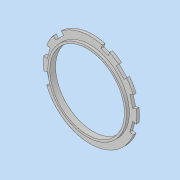
# Autodesk Inventor part: BallastTankMillOutline
Saved by Autodesk Inventor 2017.3 (Build 213256000, 256)
## iProperties
Created: 2018-07-14
Part Number: BallastTankMillOutline
Material: Generic
Document SubType Name: Modeling
Designer: Derek Wider
Density: 1 g/cm^3
Appearance: Default
Author: Derek Wider
Autodesk Inventor part; units mm, degrees
ref_plane "YZ Plane" through (0, 0, 0) normal (1, 0, 0) x (0, 1, 0)
ref_plane "XZ Plane" through (0, 0, 0) normal (0, 1, 0) x (-1, 0, 0)
ref_plane "XY Plane" through (0, 0, 0) normal (0, 0, 1) x (1, 0, 0)
sketch "Sketch1" plane through (0, 0, 0) normal (0, 0, 1) x (1, 0, 0)
  circle A0 centre (0, 0) radius 34.798
  circle A1 centre (0, 0) radius 41.275
  line L0 (38.2986, -15.3898) -> (35.2745, -14.5795)
  line L1 (35.2745, -14.5795) -> (37.8384, -5.011)
  line L2 (37.8384, -5.011) -> (40.8624, -5.8213)
  line L3 (0, 0) -> (36.5564, -9.7953) construction
  line L4 (0, 0) -> (34.798, 0) construction
  line L5 (36.5564, -9.7953) -> (39.8686, -10.6828) construction
  dimension "d0" = 69.596
  dimension "d1" = 82.55
  dimension "d2" = 15
  dimension "d3" = 9.906
  dimension "d4" = 3.429
  constraints: 12 end point, 3 point on circle, 2 coincident, 2 parallel, 1 centre point, 1 horizontal, 1 horizontal alignment, 1 midpoint, 1 perpendicular, 2 other
  measures "d1" diameter of A1
  measures "d2" angle of L3 L4
  measures "d3" distance between parallel lines of L0 L2
  measures "d4" distance of L3.end L5.end
extrude "Extrusion1" add sketch "Sketch1" along normal blind 2.54
extrude "Extrusion2" cut sketch "Sketch1" along normal blind 2.54 contours L0 L1 L2 A1 picked at (37.7926, -9.5555)
pattern_circular "Circular Pattern1" count 3 over 60 about axis through (0, 0, 0) along (0, 0, 1) of "Extrusion2"
mirror "Mirror1" about plane through (0, 0, 0) normal (1, 0, 0) of "Extrusion2", "Circular Pattern1"
sketch "Sketch2" plane through (0, 0, 0) normal (0, 0, -1) x (-1, 0, 0)
  circle A0 centre (0, 0) radius 34.798 projected
  circle A1 centre (0, 0) radius 33.02
  dimension "d12" = 66.04
  constraints: 1 centre point, 1 coincident
  measures "d12" diameter of A1
extrude "Extrusion3" add sketch "Sketch2" against normal blind 5.08
sketch "Sketch3" plane through (0, 0, 0) normal (0, 0, -1) x (-1, 0, 0)
  arc A0 (25.4726, 32.4772) -> (-25.4726, 32.4772) centre (0, 0) ccw projected
  line L0 (-17.2903, 37.4789) -> (-16.1691, 34.3986)
  line L1 (-16.1691, 34.3986) -> (-9.7247, 36.7442)
  line L2 (-9.7247, 36.7442) -> (-10.8459, 39.8245)
  line L3 (0, 0) -> (-12.9469, 35.5714) construction
  line L4 (-12.9469, 35.5714) -> (-13.8833, 38.8701) construction
  line L5 (0, 0) -> (13.6723, 0) construction
  dimension "d15" = 3.429
  dimension "d16" = 6.858
  dimension "d17" = 110
  constraints: 12 end point, 3 perpendicular, 3 point on circle, 1 horizontal, 1 midpoint
  measures "d15" distance of L3.end L4.end
  measures "d16" distance between parallel lines of L2 L0
  measures "d17" angle of L5 L3
extrude "Extrusion4" cut sketch "Sketch3" against normal blind 5.08
body "Solid1"
